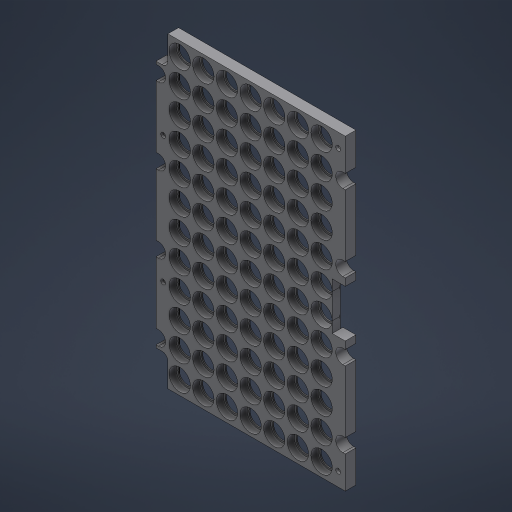
# Autodesk Inventor part: Platte1
Saved by Autodesk Inventor 2024.3 (Build 283343010, 343A)
## iProperties
Created: 2025-03-19
Part Number: Platte1
Material: Generisch
Document SubType Name: Modeling
Designer: David Lill
Density: 1 g/cm^3
Appearance: Vorgabe
Author: David Lill
Autodesk Inventor part; units mm, degrees
ref_plane "YZ Plane" through (0, 0, 0) normal (1, 0, 0) x (0, 1, 0)
ref_plane "XZ Plane" through (0, 0, 0) normal (0, 1, 0) x (-1, 0, 0)
ref_plane "XY Plane" through (0, 0, 0) normal (0, 0, 1) x (1, 0, 0)
sketch "Skizze1" plane through (0, 0, 0) normal (0, 1, 0) x (-1, 0, 0)
  line L0 (160, 0) -> (0, 0)
  line L1 (0, 0) -> (0, -260)
  line L2 (0, -260) -> (160, -260)
  line L3 (160, -260) -> (160, 0)
  circle A0 centre (140, -11.75) radius 9
  circle A1 centre (140, -54.75) radius 9
  circle A2 centre (140, -97.75) radius 9
  circle A3 centre (140, -140.75) radius 9
  circle A4 centre (140, -183.75) radius 9
  circle A5 centre (140, -226.75) radius 9
  circle A6 centre (120, -11.75) radius 9
  circle A7 centre (120, -54.75) radius 9
  circle A8 centre (120, -97.75) radius 9
  circle A9 centre (120, -140.75) radius 9
  circle A10 centre (120, -183.75) radius 9
  circle A11 centre (120, -226.75) radius 9
  circle A12 centre (100, -11.75) radius 9
  circle A13 centre (100, -54.75) radius 9
  circle A14 centre (100, -97.75) radius 9
  circle A15 centre (100, -140.75) radius 9
  circle A16 centre (100, -183.75) radius 9
  circle A17 centre (100, -226.75) radius 9
  circle A18 centre (80, -11.75) radius 9
  circle A19 centre (80, -54.75) radius 9
  circle A20 centre (80, -97.75) radius 9
  circle A21 centre (80, -140.75) radius 9
  circle A22 centre (80, -183.75) radius 9
  circle A23 centre (80, -226.75) radius 9
  circle A24 centre (60, -11.75) radius 9
  circle A25 centre (60, -54.75) radius 9
  circle A26 centre (60, -97.75) radius 9
  circle A27 centre (60, -140.75) radius 9
  circle A28 centre (60, -183.75) radius 9
  circle A29 centre (60, -226.75) radius 9
  circle A30 centre (40, -11.75) radius 9
  circle A31 centre (40, -54.75) radius 9
  circle A32 centre (40, -97.75) radius 9
  circle A33 centre (40, -140.75) radius 9
  circle A34 centre (40, -183.75) radius 9
  circle A35 centre (40, -226.75) radius 9
  circle A36 centre (20, -11.75) radius 9
  circle A37 centre (20, -54.75) radius 9
  circle A38 centre (20, -97.75) radius 9
  circle A39 centre (20, -140.75) radius 9
  circle A40 centre (20, -183.75) radius 9
  circle A41 centre (20, -226.75) radius 9
  circle A42 centre (140, -33.25) radius 9
  circle A43 centre (120, -33.25) radius 9
  circle A44 centre (100, -33.25) radius 9
  circle A45 centre (80, -33.25) radius 9
  circle A46 centre (60, -33.25) radius 9
  circle A47 centre (40, -33.25) radius 9
  circle A48 centre (20, -33.25) radius 9
  circle A49 centre (140, -76.25) radius 9
  circle A50 centre (120, -76.25) radius 9
  circle A51 centre (100, -76.25) radius 9
  circle A52 centre (80, -76.25) radius 9
  circle A53 centre (60, -76.25) radius 9
  circle A54 centre (40, -76.25) radius 9
  circle A55 centre (20, -76.25) radius 9
  circle A56 centre (140, -119.25) radius 9
  circle A57 centre (120, -119.25) radius 9
  circle A58 centre (100, -119.25) radius 9
  circle A59 centre (80, -119.25) radius 9
  circle A60 centre (60, -119.25) radius 9
  circle A61 centre (40, -119.25) radius 9
  circle A62 centre (20, -119.25) radius 9
  circle A63 centre (140, -162.25) radius 9
  circle A64 centre (120, -162.25) radius 9
  circle A65 centre (100, -162.25) radius 9
  circle A66 centre (80, -162.25) radius 9
  circle A67 centre (60, -162.25) radius 9
  circle A68 centre (40, -162.25) radius 9
  circle A69 centre (20, -162.25) radius 9
  circle A70 centre (140, -205.25) radius 9
  circle A71 centre (120, -205.25) radius 9
  circle A72 centre (100, -205.25) radius 9
  circle A73 centre (80, -205.25) radius 9
  circle A74 centre (60, -205.25) radius 9
  circle A75 centre (40, -205.25) radius 9
  circle A76 centre (20, -205.25) radius 9
  circle A77 centre (140, -248.25) radius 9
  circle A78 centre (120, -248.25) radius 9
  circle A79 centre (100, -248.25) radius 9
  circle A80 centre (80, -248.25) radius 9
  circle A81 centre (60, -248.25) radius 9
  circle A82 centre (40, -248.25) radius 9
  circle A83 centre (20, -248.25) radius 9
  line L4 (-20, 0) -> (-187, 0)
  line L5 (-207, 0) -> (-374, 0)
  circle A84 centre (140, -11.75) radius 7.5
  line L6 (155.379, -44.5989) -> (146.379, -44.5989)
  line L7 (157, -62) -> (150, -62)
  line L8 (150, -62) -> (150, -69)
  line L9 (150, -69) -> (157, -69)
  line L10 (157, -69) -> (157, -62)
  line L11 (160, -130) -> (0, -130) construction
  line L12 (157, -198) -> (150, -198)
  line L13 (150, -198) -> (150, -191)
  line L14 (150, -191) -> (157, -191)
  line L15 (157, -191) -> (157, -198)
  point P0 (80, 0)
  point P1 (153.5, -62)
  point P2 (157, -65.5)
  dimension "d0" = 160
  dimension "d1" = 260
  dimension "d4" = 18
  dimension "d7" = 43
  dimension "d10" = 20
  dimension "d16" = 21.5
  dimension "d21" = 20
  dimension "d24" = 43
  dimension "d69" = 15
  dimension "d80" = 0
  dimension "d127" = 10.75
  dimension "d129" = 7
  dimension "d130" = 7
  dimension "d132" = 3
  dimension "d134" = 10.75
  constraints: 85 centre point, 32 end point, 14 coincident, 6 horizontal, 5 midpoint, 4 parallel, 4 symmetric about line, 2 horizontal alignment, 2 perpendicular, 2 vertical, 1 equal radius, 1 vertical alignment, 164 other
  measures "d0" distance of L0.start L0.end
  measures "d1" distance of L2.end L0.start
  measures "d4" diameter of A0
  measures "d7" distance of A0.centre A1.centre
  measures "d10" distance of A0.centre A6.centre
  measures "d16" distance of A42.centre A0.centre
  measures "d21" distance of A42.centre A43.centre
  measures "d24" distance of A42.centre A49.centre
  measures "d69" diameter of A84
  measures "d80" horizontal distance of A0.centre A42.centre
  measures "d127" vertical distance of L11.start point (140, -119.25)
  measures "d129" distance of L9.end L8.end
  measures "d130" distance of L8.end L7.end
  measures "d132" distance between parallel lines of L3 L10
  measures "d134" vertical distance of point (140, -76.25) point (157, -65.5)
extrude "Extrusion1" add sketch "Skizze1" along normal blind 7 contours L3 L2 L1 L0 | A0 | A1 | A2 | A3 | A4 | A5 | A6 | A7 | A8 | A9 | A10 | A11 | A12 | A13 | A14 | A15 | A16 | A17 | A18 | A19 | A20 | A21 | A22 | A23 | A24 | A25 | A26 | A27 | A28 | A29 | A30 | A31 | A32 | A33 | A34 | A35 | A36 | A37 | A38 | A39 | A40 | A41 | A42 | A43 | A44 | A45 | A46 | A47 | A48 | A49 | A50 | A51 | A52 | A53 | A54 | A55 | A56 | A57 | A58 | A59 | A60 | A61 | A62 | A63 | A64 | A65 | A66 | A67 | A68 | A69 | A70 | A71 | A72 | A73 | A74 | A75 | A76 | A77 | A78 | A79 | A80 | A81 | A82 | A83 | A84 | L10 L9 L8 L7 | L12 L13 L14 L15
hole "Bohrung1" at (-140, 0, -11.75) at (-140, 0, -33.25) at (-140, 0, -54.75) at (-140, 0, -76.25) at (-140, 0, -97.75) at (-140, 0, -119.25) at (-140, 0, -140.75) at (-140, 0, -162.25) at (-140, 0, -183.75) at (-140, 0, -205.25) at (-140, 0, -226.75) at (-140, 0, -248.25) direction (0, 1, 0) diameter 15 end through all counterbore diameter 18 counterbore depth 6
pattern_linear "Rechteckige Anordnung1" count 7 spacing 20 along (1, 0, 0) of "Bohrung1"
sketch "Skizze2" plane through (0, 7, 0) normal (0, 1, 0) x (1, 0, 0)
  circle A0 centre (-20, 226.75) radius 9 projected
  circle A1 centre (-20, 248.25) radius 9 projected
  circle A2 centre (-20, 205.25) radius 9 projected
  circle A3 centre (-20, 162.25) radius 9 projected
  circle A4 centre (-20, 119.25) radius 9 projected
  circle A5 centre (-20, 33.25) radius 9 projected
  circle A6 centre (-20, 11.75) radius 9
  circle A7 centre (-20, 54.75) radius 9 projected
  circle A8 centre (-20, 97.75) radius 9 projected
  circle A9 centre (-20, 140.75) radius 9 projected
  circle A10 centre (-20, 183.75) radius 9 projected
  circle A11 centre (-40, 226.75) radius 9 projected
  circle A12 centre (-40, 248.25) radius 9 projected
  circle A13 centre (-40, 205.25) radius 9 projected
  circle A14 centre (-40, 162.25) radius 9 projected
  circle A15 centre (-40, 119.25) radius 9 projected
  circle A16 centre (-40, 76.25) radius 9 projected
  circle A17 centre (-40, 33.25) radius 9 projected
  circle A18 centre (-40, 11.75) radius 9 projected
  circle A19 centre (-40, 54.75) radius 9 projected
  circle A20 centre (-40, 97.75) radius 9 projected
  circle A21 centre (-40, 140.75) radius 9 projected
  circle A22 centre (-40, 183.75) radius 9 projected
  circle A23 centre (-60, 226.75) radius 9 projected
  circle A24 centre (-60, 248.25) radius 9 projected
  circle A25 centre (-60, 205.25) radius 9 projected
  circle A26 centre (-60, 162.25) radius 9 projected
  circle A27 centre (-60, 119.25) radius 9 projected
  circle A28 centre (-60, 76.25) radius 9 projected
  circle A29 centre (-60, 33.25) radius 9 projected
  circle A30 centre (-60, 11.75) radius 9 projected
  circle A31 centre (-60, 54.75) radius 9 projected
  circle A32 centre (-60, 97.75) radius 9 projected
  circle A33 centre (-60, 140.75) radius 9 projected
  circle A34 centre (-60, 183.75) radius 9 projected
  circle A35 centre (-80, 226.75) radius 9 projected
  circle A36 centre (-80, 248.25) radius 9 projected
  circle A37 centre (-80, 205.25) radius 9 projected
  circle A38 centre (-80, 162.25) radius 9 projected
  circle A39 centre (-80, 119.25) radius 9 projected
  circle A40 centre (-80, 76.25) radius 9 projected
  circle A41 centre (-80, 33.25) radius 9 projected
  circle A42 centre (-80, 11.75) radius 9 projected
  circle A43 centre (-80, 54.75) radius 9 projected
  circle A44 centre (-80, 97.75) radius 9 projected
  circle A45 centre (-80, 140.75) radius 9 projected
  circle A46 centre (-80, 183.75) radius 9 projected
  circle A47 centre (-100, 226.75) radius 9 projected
  circle A48 centre (-100, 248.25) radius 9 projected
  circle A49 centre (-100, 205.25) radius 9 projected
  circle A50 centre (-100, 162.25) radius 9 projected
  circle A51 centre (-100, 119.25) radius 9 projected
  circle A52 centre (-100, 76.25) radius 9 projected
  circle A53 centre (-100, 33.25) radius 9 projected
  circle A54 centre (-100, 11.75) radius 9 projected
  circle A55 centre (-100, 54.75) radius 9 projected
  circle A56 centre (-100, 97.75) radius 9 projected
  circle A57 centre (-100, 140.75) radius 9 projected
  circle A58 centre (-100, 183.75) radius 9 projected
  circle A59 centre (-120, 226.75) radius 9 projected
  circle A60 centre (-120, 248.25) radius 9 projected
  circle A61 centre (-120, 205.25) radius 9 projected
  circle A62 centre (-120, 162.25) radius 9 projected
  circle A63 centre (-120, 119.25) radius 9 projected
  circle A64 centre (-120, 76.25) radius 9 projected
  circle A65 centre (-120, 33.25) radius 9 projected
  circle A66 centre (-120, 11.75) radius 9 projected
  circle A67 centre (-120, 54.75) radius 9 projected
  circle A68 centre (-120, 97.75) radius 9 projected
  circle A69 centre (-120, 140.75) radius 9 projected
  circle A70 centre (-120, 183.75) radius 9 projected
  circle A71 centre (-140, 226.75) radius 9 projected
  circle A72 centre (-140, 183.75) radius 9 projected
  circle A73 centre (-140, 140.75) radius 9 projected
  circle A74 centre (-140, 97.75) radius 9 projected
  circle A75 centre (-140, 54.75) radius 9 projected
  circle A76 centre (-140, 11.75) radius 9 projected
  circle A77 centre (-140, 33.25) radius 9 projected
  circle A78 centre (-140, 76.25) radius 9 projected
  circle A79 centre (-140, 119.25) radius 9 projected
  circle A80 centre (-140, 162.25) radius 9 projected
  circle A81 centre (-140, 205.25) radius 9 projected
  circle A82 centre (-140, 248.25) radius 9 projected
  line L0 (0, 0) -> (0, 260) projected
  line L1 (-160, 0) -> (0, 0) projected
  line L2 (-160, 260) -> (-160, 0) projected
  line L3 (0, 260) -> (-160, 260) projected
  line L4 (-160, 0) -> (0, 0) projected
  line L5 (-150, 0) -> (-150, 55)
  arc A83 (-150, 55) -> (-155, 60) centre (-155, 55) ccw
  line L6 (-155, 60) -> (-160, 60)
  line L7 (-160, 260) -> (-160, 0) projected
  line L8 (-160, 0) -> (0, 0) projected
  line L9 (0, 0) -> (0, 260) projected
  line L10 (-160, 260) -> (-160, 0) projected
  line L11 (0, 260) -> (-160, 260) projected
  line L12 (-160, 25) -> (-155, 25)
  arc A84 (-150, 20) -> (-155, 25) centre (-155, 20) ccw
  line L13 (0, 130) -> (-160, 130)
  line L14 (-150, 260) -> (-150, 205)
  arc A85 (-155, 200) -> (-150, 205) centre (-155, 205) ccw
  line L15 (-155, 200) -> (-160, 200)
  line L16 (-160, 235) -> (-155, 235)
  arc A86 (-155, 235) -> (-150, 240) centre (-155, 240) ccw
  circle A87 centre (-20, 11.75) radius 9 projected
  line L17 (-143.0414, 85.25) -> (-151, 85.25)
  arc A88 (-151, 85.25) -> (-151, 67.25) centre (-151, 76.25) ccw
  line L18 (-151, 67.25) -> (-143.0414, 67.25)
  arc A89 (-143.0414, 85.25) -> (-143.0414, 67.25) centre (-140, 76.25) ccw
  line L19 (-143.0414, 174.75) -> (-151, 174.75)
  arc A90 (-151, 192.75) -> (-151, 174.75) centre (-151, 183.75) ccw
  line L20 (-151, 192.75) -> (-143.0414, 192.75)
  arc A91 (-143.0414, 192.75) -> (-143.0414, 174.75) centre (-140, 183.75) ccw
  circle A92 centre (-154, 76.25) radius 4
  circle A93 centre (-154, 183.75) radius 4
  line L21 (-80, 260) -> (-80, 0)
  line L22 (0, 232.75) -> (-2, 232.75)
  arc A94 (-2, 232.75) -> (-2, 220.75) centre (-2, 226.75) ccw
  line L23 (-2, 220.75) -> (0, 220.75)
  line L24 (0, 168.25) -> (-2, 168.25)
  arc A95 (-2, 168.25) -> (-2, 156.25) centre (-2, 162.25) ccw
  line L25 (-2, 156.25) -> (0, 156.25)
  line L26 (-160, 168.25) -> (-158, 168.25)
  arc A96 (-158, 156.25) -> (-158, 168.25) centre (-158, 162.25) ccw
  line L27 (-158, 156.25) -> (-160, 156.25)
  line L28 (0, 27.25) -> (-2, 27.25)
  arc A97 (-2, 39.25) -> (-2, 27.25) centre (-2, 33.25) ccw
  line L29 (-2, 39.25) -> (0, 39.25)
  line L30 (0, 91.75) -> (-2, 91.75)
  arc A98 (-2, 103.75) -> (-2, 91.75) centre (-2, 97.75) ccw
  line L31 (-2, 103.75) -> (0, 103.75)
  arc A99 (-158, 91.75) -> (-158, 103.75) centre (-158, 97.75) ccw
  line L32 (-160, 91.75) -> (-158, 91.75)
  line L33 (-158, 103.75) -> (-160, 103.75)
  line L34 (-16.9586, 20.75) -> (-9, 20.75)
  arc A100 (-9, 2.75) -> (-9, 20.75) centre (-9, 11.75) ccw
  line L35 (-9, 2.75) -> (-16.9586, 2.75)
  arc A101 (-16.9586, 2.75) -> (-16.9586, 20.75) centre (-20, 11.75) ccw
  circle A102 centre (-6, 11.75) radius 4
  arc A103 (-9, 239.25) -> (-9, 257.25) centre (-9, 248.25) ccw
  line L36 (-9, 257.25) -> (-16.9586, 257.25)
  arc A104 (-16.9586, 239.25) -> (-16.9586, 257.25) centre (-20, 248.25) ccw
  line L37 (-16.9586, 239.25) -> (-9, 239.25)
  circle A105 centre (-6, 248.25) radius 4
  line L38 (-160, 232.75) -> (-158, 232.75)
  arc A106 (-158, 220.75) -> (-158, 232.75) centre (-158, 226.75) ccw
  line L39 (-158, 220.75) -> (-160, 220.75)
  arc A107 (-158, 27.25) -> (-158, 39.25) centre (-158, 33.25) ccw
  line L40 (-160, 27.25) -> (-158, 27.25)
  line L41 (-158, 39.25) -> (-160, 39.25)
  line L42 (-11, 199.5) -> (-3, 199.5)
  line L43 (-3, 199.5) -> (-3, 179.5)
  line L44 (-3, 179.5) -> (-11, 179.5)
  line L45 (-11, 179.5) -> (-11, 199.5)
  line L46 (-11, 60.5) -> (-3, 60.5)
  line L47 (-3, 60.5) -> (-3, 80.5)
  line L48 (-3, 80.5) -> (-11, 80.5)
  line L49 (-11, 80.5) -> (-11, 60.5)
  line L50 (-156.36, 69) -> (-149.36, 69)
  line L51 (-149.36, 69) -> (-149.36, 62)
  line L52 (-149.36, 62) -> (-156.36, 62)
  line L53 (-156.36, 62) -> (-156.36, 69)
  line L54 (-156.36, 191) -> (-149.36, 191)
  line L55 (-149.36, 191) -> (-149.36, 198)
  line L56 (-149.36, 198) -> (-156.36, 198)
  line L57 (-156.36, 198) -> (-156.36, 191)
  point P0 (-160, 60)
  point P1 (0, 130)
  point P2 (-150, 260)
  point P3 (-160, 200)
  point P4 (-160, 235)
  point P5 (-160, 25)
  point P6 (0, 27.25)
  point P7 (0, 39.25)
  point P8 (0, 103.75)
  point P9 (-4, 226.75)
  point P10 (-4, 162.25)
  point P11 (-4, 33.25)
  point P12 (-4, 97.75)
  point P13 (-156, 226.75)
  point P14 (-156, 162.25)
  point P15 (-156, 97.75)
  point P16 (-156, 33.25)
  point P17 (-7, 199.5)
  point P18 (-7, 179.5)
  point P19 (-3, 189.5)
  point P20 (-11, 189.5)
  point P21 (-152.86, 69)
  point P22 (-149.36, 65.5)
  dimension "d83" = 10
  dimension "d84" = 5
  dimension "d85" = 60
  dimension "d101" = 25
  dimension "d119" = 8
  dimension "d121" = 6
  dimension "d124" = 33.25
  dimension "d125" = 64.5
  dimension "d126" = 6
  dimension "d135" = 9.5
  dimension "d136" = 2
  dimension "d142" = 6
  dimension "d143" = 4
  dimension "d144" = 4
  dimension "d160" = 8
  dimension "d162" = 3
  dimension "d165" = 20
  dimension "d166" = 5.75
  dimension "d169" = 7
  dimension "d170" = 7
  dimension "d171" = 3.64
  dimension "d172" = 10.75
  constraints: 107 centre point, 96 end point, 68 symmetric about line, 40 point on circle, 14 tangent, 11 midpoint, 9 point on line, 7 horizontal, 7 parallel, 7 perpendicular, 6 coincident, 6 equal radius, 6 horizontal alignment, 2 vertical, 2 vertical alignment, 1 concentric, 14 other
  measures "d83" distance between parallel lines of L2 L5
  measures "d84" radius of A83
  measures "d85" distance between parallel lines of L6 L4
  measures "d101" distance between parallel lines of L4 L12
  measures "d119" diameter of A92
  measures "d121" distance from line of L2 A92.centre
  measures "d124" distance from line of L11 point (-2, 226.75)
  measures "d125" distance of point (-2, 226.75) point (-2, 162.25)
  measures "d126" radius of A94
  measures "d135" radius of A89
  measures "d136" distance from line of L0 point (-2, 226.75)
  measures "d142" distance from line of L9 A102.centre
  measures "d143" distance from line of L0 point (-4, 226.75)
  measures "d144" distance from line of L0 point (-4, 162.25)
  measures "d160" distance of point (-3, 189.5) point (-11, 189.5)
  measures "d162" distance from line of L9 L42.end
  measures "d165" distance of L42.end L43.end
  measures "d166" distance from line of A2.centre L42
  measures "d169" distance from line of L52 point (-152.86, 69)
  measures "d170" distance of L50.start L50.end
  measures "d171" distance between parallel lines of L10 L53
  measures "d172" vertical distance of A89.centre point (-149.36, 65.5)
extrude "Extrusion2" cut sketch "Skizze2" against normal blind 10 contours L14 A86 L16 L2 L3 | L12 A84 L5 L1 L2
extrude "Extrusion4" cut sketch "Skizze2" against normal up to surface (7 mm away) contours L0 L23 A94 L22 | L38 A106 L39 L2 | L0 L25 A95 L24 | L26 A96 L27 L2 | L0 L30 A98 L31 | L33 A99 L32 L2 | L0 L28 A97 L29 | L41 A107 L40 L2
hole "Bohrung4" at (-2, 7, -226.75) at (-2, 7, -162.25) at (-158, 7, -162.25) at (-2, 7, -33.25) at (-2, 7, -97.75) at (-6, 7, -248.25) at (-6, 7, -11.75) at (-154, 7, -183.75) at (-154, 7, -76.25) direction (0, -1, 0) diameter 4 end through all counterbore diameter 6 counterbore depth 5
sketch "Skizze3" plane through (0, 7, 0) normal (0, 1, 0) x (1, 0, 0)
  point P0 (0, 0)
sketch "Skizze4" plane through (0, 7, 0) normal (0, 1, 0) x (1, 0, 0)
  line L0 (-150, 0) -> (0, 0) projected
  line L1 (0, 260) -> (-150, 260) projected
  line L2 (-16, 258) -> (-144, 258)
  line L3 (-144, 2) -> (-16, 2)
  arc A0 (-16, 2) -> (-11, 7) centre (-16, 7) ccw
  line L4 (-11, 7) -> (-11, 253)
  arc A1 (-11, 253) -> (-16, 258) centre (-16, 253) ccw
  circle A2 centre (-20, 248.25) radius 7.5 projected
  arc A3 (-149, 7) -> (-144, 2) centre (-144, 7) ccw
  arc A4 (-144, 258) -> (-149, 253) centre (-144, 253) ccw
  line L5 (-149, 253) -> (-149, 7)
  circle A5 centre (-140, 248.25) radius 7.5 projected
  arc A6 (-2, 103.75) -> (-2, 91.75) centre (-2, 97.75) ccw projected
  line L6 (-2, 103.75) -> (0, 103.75) projected
  line L7 (0, 91.75) -> (-2, 91.75) projected
  line L8 (0, 39.25) -> (0, 91.75) projected
  line L9 (0, 103.75) -> (0, 156.25) projected
  line L10 (0, 156.25) -> (-2, 156.25) projected
  arc A7 (-2, 168.25) -> (-2, 156.25) centre (-2, 162.25) ccw projected
  line L11 (-2, 168.25) -> (0, 168.25) projected
  line L12 (0, 168.25) -> (0, 220.75) projected
  line L13 (0, 232.75) -> (0, 260) projected
  line L14 (-2, 232.75) -> (0, 232.75) projected
  arc A8 (-2, 232.75) -> (-2, 220.75) centre (-2, 226.75) ccw projected
  line L15 (0, 220.75) -> (-2, 220.75) projected
  line L16 (0, 0) -> (0, 27.25) projected
  line L17 (-2, 39.25) -> (0, 39.25) projected
  arc A9 (-2, 39.25) -> (-2, 27.25) centre (-2, 33.25) ccw projected
  line L18 (0, 27.25) -> (-2, 27.25) projected
  line L19 (-150, 260) -> (-150, 240) projected
  arc A10 (-155, 235) -> (-150, 240) centre (-155, 240) ccw projected
  line L20 (-155, 235) -> (-160, 235) projected
  arc A11 (-158, 220.75) -> (-158, 232.75) centre (-158, 226.75) ccw projected
  line L21 (-160, 220.75) -> (-160, 168.25) projected
  line L22 (-158, 220.75) -> (-160, 220.75) projected
  line L23 (-160, 232.75) -> (-158, 232.75) projected
  line L24 (-160, 235) -> (-160, 232.75) projected
  line L25 (-158, 156.25) -> (-160, 156.25) projected
  arc A12 (-158, 156.25) -> (-158, 168.25) centre (-158, 162.25) ccw projected
  line L26 (-160, 168.25) -> (-158, 168.25) projected
  line L27 (-160, 156.25) -> (-160, 103.75) projected
  line L28 (-160, 103.75) -> (-158, 103.75) projected
  arc A13 (-158, 91.75) -> (-158, 103.75) centre (-158, 97.75) ccw projected
  line L29 (-158, 91.75) -> (-160, 91.75) projected
  line L30 (-160, 91.75) -> (-160, 39.25) projected
  line L31 (-150, 20) -> (-150, 0) projected
  arc A14 (-150, 20) -> (-155, 25) centre (-155, 20) ccw projected
  line L32 (-160, 25) -> (-155, 25) projected
  line L33 (-160, 27.25) -> (-160, 25) projected
  line L34 (-158, 27.25) -> (-160, 27.25) projected
  arc A15 (-158, 27.25) -> (-158, 39.25) centre (-158, 33.25) ccw projected
  line L35 (-160, 39.25) -> (-158, 39.25) projected
  circle A16 centre (-6, 11.75) radius 3 projected
  circle A17 centre (-6, 248.25) radius 3 projected
  circle A18 centre (-154, 76.25) radius 3 projected
  circle A19 centre (-154, 183.75) radius 3 projected
  line L36 (-11, 110) -> (0, 110)
  line L37 (-11, 150) -> (0, 150)
  point P0 (-154.75, 102.7936)
  point P1 (-154.75, 157.2064)
  point P2 (-154.75, 38.2936)
  point P3 (-154.75, 73.3453)
  point P4 (-154.75, 79.1547)
  point P5 (-154.75, 92.7064)
  point P6 (-150, 20)
  point P7 (-154.75, 28.2064)
  point P8 (-154.75, 231.7936)
  point P9 (-154.75, 167.2936)
  point P10 (-154.75, 180.8453)
  point P11 (-154.75, 186.6547)
  point P12 (-154.75, 221.7064)
  point P13 (-150, 252)
  point P14 (-5.25, 251.1547)
  point P15 (-3, 248.25)
  point P16 (-3, 232.6661)
  point P17 (-3, 220.8339)
  point P18 (-3, 168.1661)
  point P19 (-3, 156.3339)
  point P20 (-3, 103.6661)
  point P21 (-3, 91.8339)
  point P22 (-3, 39.1661)
  point P23 (-3, 27.3339)
  point P24 (-3, 11.75)
  point P25 (-5.25, 8.8453)
  point P26 (-150, 8)
  point P27 (-11, 130)
  dimension "d180" = 2
  dimension "d181" = 2
  dimension "d182" = 5
  dimension "d184" = 9
  dimension "d185" = 9
  dimension "d190" = 40
  dimension "d191" = 20
  constraints: 12 end point, 8 point on circle, 8 tangent, 4 centre point, 4 point on line, 3 equal radius, 2 parallel, 2 perpendicular, 2 vertical, 1 midpoint
  measures "d180" distance between parallel lines of L1 L2
  measures "d181" distance between parallel lines of L0 L3
  measures "d182" radius of A1
  measures "d184" distance from line of L5 A5.centre
  measures "d185" distance from line of A2.centre L4
  measures "d190" distance between parallel lines of L37 L36
  measures "d191" distance from line of point (-11, 130) L36
extrude "Extrusion6" add sketch "Skizze4" along normal blind 2 contours L31 A14 L32 L33 L34 A15 L35 L30 L29 A13 L28 L27 L25 A12 L26 L21 L22 A11 L23 L24 L20 A10 L19 L1 L13 L14 A8 L15 L12 L11 A7 L10 L9 L37 L4 A1 L2 A4 L5 A3 L3 A0 L36 L6 A6 L7 L8 L17 A9 L18 L16 L0 | A16 | A17 | A18 | A19
extrude "Extrusion7" cut sketch "Skizze4" against normal through all contours L36 L4 L37 L9
equation "\"d16\" = 0.5 * d7"
equation "\"d21\" = d10"
equation "\"d24\" = d7"
